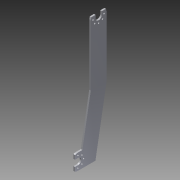
# Autodesk Inventor part: 09
Saved by Autodesk Inventor 2013 (Build 170138000, 138)
## iProperties
Created: 2014-03-10
Part Number: 09
Material: アルミニウム 6061
Document SubType Name: Modeling
Designer: andou
Density: 1 g/cm^3
Author: andou
Title: Dual_Link_Flame(right)
Autodesk Inventor part; units mm, degrees
ref_plane "YZ Plane" through (0, 0, 0) normal (1, 0, 0) x (0, 1, 0)
ref_plane "XZ Plane" through (0, 0, 0) normal (0, 1, 0) x (-1, 0, 0)
ref_plane "XY Plane" through (0, 0, 0) normal (0, 0, 1) x (1, 0, 0)
sketch "スケッチ1" plane through (0, 0, 0) normal (1, 0, 0) x (0, 1, 0)
  line L0 (-20, 80) -> (20, 80)
  line L1 (20, 80) -> (20, -80)
  line L2 (20, -80) -> (-20, -80)
  line L3 (-20, -80) -> (-20, 80)
  point P0 (0, 0)
  dimension "d0" = 160
  dimension "d2" = 40
  dimension "d3" = 20
  dimension "d4" = 80
  constraints: 8 end point, 2 parallel, 1 horizontal, 1 perpendicular
  measures "d0" distance of L2.end L0.start
  measures "d2" distance of L1.end L2.end
  measures "d3" distance from line of L3 point (0, 0)
  measures "d4" distance from line of point (0, 0) L2
extrude "押し出し1" add sketch "スケッチ1" along normal blind 2
sketch "スケッチ2" plane through (2, 0, 0) normal (1, 0, 0) x (0, 0, -1)
  line L0 (80, -20) -> (80, 20) projected
  line L1 (80, 20) -> (-80, 20) projected
  line L2 (-80, 20) -> (80, 20)
  line L3 (80, 20) -> (80, 18)
  line L4 (80, 18) -> (-80, 18)
  line L5 (-80, 18) -> (-80, 20)
  point P0 (0, 0)
  dimension "d7" = 2
  constraints: 8 end point, 2 parallel, 1 horizontal, 1 perpendicular, 1 point on line
  measures "d7" distance between parallel lines of L2 L4
extrude "押し出し2" add sketch "スケッチ2" along normal blind 20
sketch "スケッチ3" plane through (0, 0, 0) normal (-1, 0, 0) x (0, 0, 1)
  line L0 (80, -20) -> (80, 20) projected
  line L1 (80, 20) -> (-80, 20) projected
  line L2 (-80, 20) -> (-80, -20) projected
  line L3 (-80, -20) -> (80, -20) projected
  line L4 (-60, -20) -> (-60, -10.5796)
  line L5 (-60, -10.5796) -> (0, 0)
  line L6 (0, 0) -> (80, 0)
  line L7 (80, 0) -> (80, 20)
  line L8 (-80, 5.8938) -> (0, 20)
  point P0 (0, 0)
  dimension "d11" = 20
  dimension "d12" = 10
  dimension "d13" = 10
  dimension "d14" = 20
  dimension "d15" = 160
  dimension "d17" = 80
  dimension "d18" = 80
  constraints: 10 end point, 3 perpendicular, 3 point on line, 1 midpoint
  measures "d11" distance between parallel lines of L2 L4
  measures "d12" angle of L1 L8
  measures "d13" angle of L6 L5
  measures "d14" distance between parallel lines of L1 L6
  measures "d15" distance between parallel lines of L2 L7
  measures "d17" distance of L7.end L8.end
  measures "d18" distance of L6.end L5.end
extrude "押し出し3" cut sketch "スケッチ3" against normal blind 20 contours L6 L5 L4 L3 L2 L8 L1 L0 keep common part
sketch "スケッチ6" plane through (0, 0, 0) normal (-1, 0, 0) x (0, 0, 1)
  line L0 (-60, -10.5796) -> (-60, -20) projected
  line L1 (0, 0) -> (-60, -10.5796) projected
  line L2 (80, 0) -> (0, 0) projected
  line L3 (80, 0) -> (80, 20) projected
  line L4 (80, 20) -> (0, 20) projected
  line L5 (-80, 5.8938) -> (0, 20) projected
  line L6 (-80, 5.8938) -> (-80, -20) projected
  line L7 (-80, -20) -> (-60, -20) projected
  arc A0 (-66, -16) -> (-74, -16) centre (-70, -16) ccw
  arc A1 (76, 14) -> (76, 6) centre (76, 10) ccw
  line L8 (-74, -16) -> (-74, -20)
  line L9 (-66, -16) -> (-66, -20)
  line L10 (76, 14) -> (80, 14)
  line L11 (76, 6) -> (80, 6)
  arc A2 (-60.8348, -20) -> (-60, -16) centre (-70, -16) ccw
  arc A3 (-80, -16) -> (-79.1652, -20) centre (-70, -16) ccw
  arc A4 (76, 0) -> (80, 0.8348) centre (76, 10) ccw
  arc A5 (80, 19.1652) -> (76, 20) centre (76, 10) ccw
  point P0 (0, 0)
  dimension "d37" = 8
  dimension "d39" = 8
  dimension "d40" = 4
  dimension "d41" = 4
  dimension "d42" = 10
  dimension "d43" = 10
  constraints: 12 point on circle, 12 point on line, 8 end point, 6 centre point, 6 tangent, 3 perpendicular, 2 coincident, 2 concentric, 1 parallel
  measures "d37" diameter of A0
  measures "d39" diameter of A1
  measures "d40" distance from line of A0.centre L7
  measures "d41" distance from line of A1.centre L3
  measures "d42" distance from line of L4 A1.centre
  measures "d43" distance from line of L6 A0.centre
extrude "押し出し6" cut sketch "スケッチ6" against normal blind 11 contours L0 A2 L7 L9 A0 L8 A3 L6 L5 L4 A5 L3 L10 A1 L11 A4 L2 L1 keep common part
sketch "スケッチ7" plane through (0, 0, 0) normal (-1, 0, 0) x (0, 0, 1)
  arc A0 (80, 19.1652) -> (76, 20) centre (76, 10) ccw projected
  arc A1 (-80, -16) -> (-79.1652, -20) centre (-70, -16) ccw projected
  line L0 (-79.1652, -20) -> (-74, -20) projected
  line L1 (80, 0.8348) -> (80, 6) projected
  circle A2 centre (76, 3) radius 1
  circle A3 centre (-77, -16) radius 1
  point P0 (0, 0)
  dimension "d46" = 2
  dimension "d48" = 7
  dimension "d49" = 4
  dimension "d50" = 4
  dimension "d51" = 7
  constraints: 2 centre point, 1 equal radius
  measures "d46" diameter of A2
  measures "d48" distance of A0.centre A2.centre
  measures "d49" distance from line of L1 A2.centre
  measures "d50" distance from line of A3.centre L0
  measures "d51" distance of A1.centre A3.centre
hole "穴1" at (0, -16, -77) at (0, 3, 76) direction (1, 0, 0) diameter 2 end through all
pattern_circular "円形状パターン1" count 5 over 180 about axis through (0, -16, -70) along (1, 0, 0) of "穴1"
pattern_circular "円形状パターン2" count 5 over 180 about axis through (0, 10, 76) along (1, 0, 0) of "穴1"
sketch "スケッチ11" plane through (2, 18, 80) normal (0, -1, 0) x (1, 0, 0)
  line L0 (9, 0) -> (9, -91.3426) projected
  line L1 (0, 0) -> (9, 0) projected
  line L2 (0, -4) -> (0, 0) projected
  line L3 (0, -91.3426) -> (0, -4) projected
  line L4 (9, -91.3426) -> (0, -91.3426) projected
  point P0 (-2, -80)
extrude "押し出し10" cut sketch "スケッチ11" against normal blind 2
